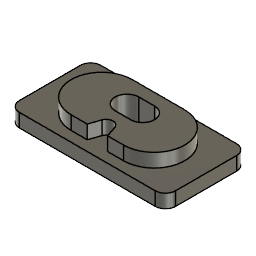
Heater cable spacer (Autodesk Fusion 360 design; units mm, degrees)
Autodesk Fusion 360 part; units mm, degrees
sketch "Sketch1" plane through (0, 0, 0) normal (0, 0, 1) x (1, 0, 0)
  line L0 (-3.85, 0) -> (3.85, 0) construction
  line L1 (-3.85, 0) -> (-8.35, 0) construction
  line L2 (3.85, 0) -> (8.35, 0) construction
  line L3 (0, 0) -> (0, -3.2) construction
  line L4 (-3.85, -4.5) -> (3.85, -4.5)
  line L5 (3.85, 4.5) -> (-3.85, 4.5)
  arc A0 (-3.85, 4.5) -> (-3.85, -4.5) centre (-3.85, 0) ccw
  arc A1 (3.85, -4.5) -> (3.85, 4.5) centre (3.85, 0) ccw
  line L6 (-0.9465, -2.8772) -> (-1.5, -4.5)
  line L7 (0.9465, -2.8772) -> (1.5, -4.5)
  arc A2 (0.9465, -2.8772) -> (-0.9465, -2.8772) centre (0, -3.2) ccw
  line L8 (11.5, -6) -> (-11.5, -6)
  line L9 (-11.5, -6) -> (-11.5, 6)
  line L10 (-11.5, 6) -> (11.5, 6)
  line L11 (11.5, 6) -> (11.5, -6)
  line L12 (11.5, -6) -> (-11.5, 6) construction
  line L13 (-11.5, -6) -> (11.5, 6) construction
  line L14 (-1.15, 2.75) -> (1.15, 2.75)
  line L15 (1.15, -0.75) -> (-1.15, -0.75)
  arc A3 (1.15, -0.75) -> (1.15, 2.75) centre (1.15, 1) ccw
  arc A4 (-1.15, 2.75) -> (-1.15, -0.75) centre (-1.15, 1) ccw
  line L16 (-1.15, 1) -> (1.15, 1)
  dimension "d1" = 9
  dimension "d2" = 16.7
  dimension "d3" = 2
  dimension "d4" = 3.2
  dimension "d5" = 3
  dimension "d6" = 12
  dimension "d7" = 23
  dimension "d12" = 3.5
  dimension "d13" = 2.3
  dimension "d20" = 1
  constraint equal A0 A1
  constraint horizontal L0
  constraint coincident L0.end L2.start
  constraint coincident L0.start L1.start
  constraint coincident L1.end A0
  constraint parallel L0 L1
  constraint coincident L2.end A1
  constraint parallel L0 L2
  constraint midpoint L0 L3.start
  constraint perpendicular L0 L3
  constraint coincident L3.end A2.centre
  constraint tangent L4 A1
  constraint horizontal L4
  constraint tangent L5 A0
  constraint parallel L0 L5
  constraint coincident L4 L6.end
  constraint coincident L4 L7.end
  constraint tangent L7 A2
  constraint tangent L6 A2
  constraint symmetric L3 L6 L7
  constraint coincident L3.start origin
  constraint horizontal L8
  constraint perpendicular L8 L9
  constraint parallel L8 L10
  constraint parallel L9 L11
  constraint coincident L12 L3.start
  constraint coincident L13 L3.start
  constraint equal A3 A4
  constraint tangent L14 A3
  constraint horizontal L14
  constraint tangent L15 A4
  constraint perpendicular L3 L15
  constraint symmetric L3 A3 A4
  constraint coincident A4.centre L16.start
  constraint coincident A3.centre L16.end
  measures "d1" diameter of A0
  measures "d2" distance of L1.end L2.end
  measures "d3" diameter of A2
  measures "d4" distance of L3.start L3.end
  measures "d5" distance of L6.end L7.end
  measures "d6" distance of L8 L10
  measures "d7" distance of L8.start L8.end
  measures "d12" distance of L14 L15
  measures "d13" distance of A4.centre A3.centre
  measures "d20" distance of L3.start L16
extrude "Extrude1" add sketch "Sketch1" against normal blind 2 contours L4 L5 A0 A1 L6 L7 A2 | L4 L6 L7 A2 | L8 L9 L10 L11 | L14 L15 A3 A4
extrude "Extrude2" add sketch "Sketch1" along normal blind 2 contours L4 L5 A0 A1 L6 L7 A2 | L14 L15 A3 A4
extrude "Extrude3" cut sketch "Sketch1" along normal up to surface (2 mm away) and the other way up to surface (2 mm away) contours L14 L15 A3 A4
fillet "Fillet1" radius 1.5 4 edges at (11.5, -6, -1) (-11.5, -6, -1) (-11.5, 6, -1) (11.5, 6, -1)
equation "d6 = 9 mm + 3 mm"
equation "d13 = 5.8 mm - 3.5 mm"
named bodies: "Cable_spacer"
